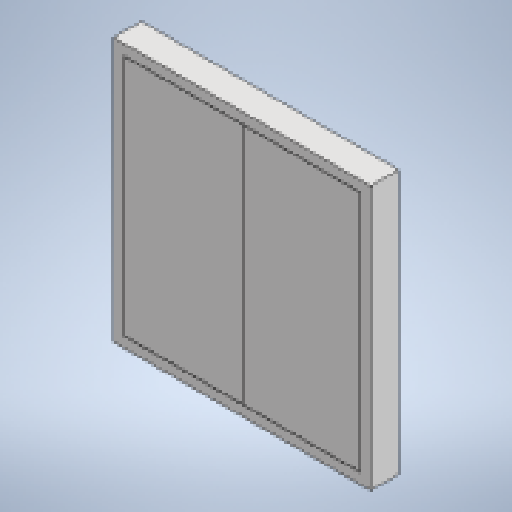
# Autodesk Inventor part: BSH 0 foudation
Saved by Autodesk Inventor 2025 (Build 290162010, 162A)
## iProperties
Created: 2024-08-27
Part Number: BSH 0 foudation
Material: Generic
Document SubType Name: Modeling
Designer: DELL
Density: 1 g/cm^3
Appearance: Default
Author: DELL
Autodesk Inventor part; units mm, degrees
ref_plane "YZ Plane" through (0, 0, 0) normal (1, 0, 0) x (0, 1, 0)
ref_plane "XZ Plane" through (0, 0, 0) normal (0, 1, 0) x (-1, 0, 0)
ref_plane "XY Plane" through (0, 0, 0) normal (0, 0, 1) x (1, 0, 0)
sketch "Sketch1" plane through (0, 0, 0) normal (0, 1, 0) x (-1, 0, 0)
  line L0 (15.7014, 4425) -> (-15.7014, 4425)
  line L1 (4425, 4550) -> (-4425, 4550)
  line L2 (-4425, 4550) -> (-4425, -4550)
  line L3 (-4425, -4550) -> (4425, -4550)
  line L4 (4425, -4550) -> (4425, 4550)
  line L5 (4425, 4550) -> (-4425, -4550) construction
  line L6 (-4425, 4550) -> (4425, -4550) construction
  line L7 (-4825, 4950) -> (4825, 4950)
  line L8 (4825, 4950) -> (4825, -4950)
  line L9 (4825, -4950) -> (-4825, -4950)
  line L10 (-4825, -4950) -> (-4825, 4950)
  point P0 (0, 0)
  point P1 (0, 0)
  dimension "d0" = 8850
  dimension "d1" = 9100
  dimension "d3" = 400
  constraints: 22 end point, 4 parallel, 2 horizontal, 2 midpoint, 2 perpendicular, 1 coincident, 3 other
  measures "d0" distance of L3.end L2.end
  measures "d1" distance of L2.end L1.end
  measures "d3" distance between parallel lines of L1 L7
extrude "Extrusion1" add sketch "Sketch1" along normal blind 650 and the other way blind 400
sketch "Sketch4" plane through (0, -400, 0) normal (0, -1, 0) x (1, 0, 0)
  line L0 (-4825, -4950) -> (4825, -4950) projected
  line L1 (4825, -4950) -> (4825, 4950) projected
  line L2 (4825, 4950) -> (-4825, 4950) projected
  line L3 (-4825, 4950) -> (-4825, -4950) projected
  line L4 (-4425, -4550) -> (-4425, 4550) projected
  line L5 (-4425, 4550) -> (4425, 4550) projected
  line L6 (4425, 4550) -> (4425, -4550) projected
  line L7 (4425, -4550) -> (-4425, -4550) projected
  point P0 (0, 0)
extrude "Extrusion3" add sketch "Sketch4" along normal blind 10 contours L4 L5 L6 L7
sketch "Sketch5" plane through (0, 0, 0) normal (0, 1, 0) x (-1, 0, 0)
  line L0 (-4825, -4950) -> (4825, -4950) projected
  line L1 (4825, -4950) -> (4825, 4950) projected
  line L2 (4825, 4950) -> (-4825, 4950) projected
  line L3 (-4825, 4950) -> (-4825, -4950) projected
  line L4 (4425, 4550) -> (4425, -4550) projected
  line L5 (4425, -4550) -> (-4425, -4550) projected
  line L6 (-4425, -4550) -> (-4425, 4550) projected
  line L7 (-4425, 4550) -> (4425, 4550) projected
  line L8 (5, 4550) -> (5, -4550)
  point P0 (0, 0)
  dimension "d21" = 4420
  constraints: 2 end point, 2 point on line, 1 perpendicular
  measures "d21" distance between parallel lines of L4 L8
extrude "Extrusion4" add sketch "Sketch5" against normal up to surface (400 mm away) contours L4 L5 L8 L7
sketch "Sketch6" plane through (0, 650, 0) normal (0, 1, 0) x (1, 0, 0)
  line L0 (4825, 4950) -> (-4825, 4950) projected
  line L1 (-4825, 4950) -> (-4825, -4950) projected
  line L2 (-4825, -4950) -> (4825, -4950) projected
  line L3 (4825, -4950) -> (4825, 4950) projected
  line L4 (-4425, -4550) -> (-4425, 4550) projected
  line L5 (-4425, 4550) -> (4425, 4550) projected
  line L6 (4425, 4550) -> (4425, -4550) projected
  line L7 (4425, -4550) -> (-4425, -4550) projected
  line L8 (1295, -4950) -> (1295, -4550)
  line L9 (2395, -4950) -> (2395, -4550)
  line L10 (-5, -4550) -> (-5, 4550) projected
  point P0 (0, 0)
  dimension "d24" = 1100
  dimension "d25" = 1300
  constraints: 4 end point, 4 point on line, 2 perpendicular
  measures "d24" distance between parallel lines of L9 L8
  measures "d25" distance between parallel lines of L8 L10
extrude "Extrusion5" cut sketch "Sketch6" against normal blind 10 contours L2 L8 L7 L9
sketch "Sketch7" plane through (1295, 650, 4950) normal (1, 0, 0) x (0, 0, -1)
  line L0 (0, -1050) -> (0, 0) projected
  line L1 (9900, 0) -> (0, 0) projected
  line L2 (9900, -1050) -> (9900, 0) projected
  line L3 (0, -1050) -> (9900, -1050) projected
  line L4 (9500, -1050) -> (400, -1050) projected
  line L5 (9500, -650) -> (9500, -1050) projected
  line L6 (400, -650) -> (9500, -650) projected
  line L7 (400, -1050) -> (400, -650) projected
  line L8 (400, 0) -> (400, -650) projected
  line L9 (400, 0) -> (1200, -150)
  line L10 (1200, -150) -> (1200, -650)
  line L11 (1200, -150) -> (2700, -150)
  line L12 (2700, -150) -> (2700, -650)
  point P0 (4950, -650)
  point P1 (400, -1050)
  dimension "d42" = 10.62
  dimension "d43" = 1500
  dimension "d48" = 800
  dimension "d55" = 900
  constraints: 8 end point, 2 point on line, 1 horizontal, 1 perpendicular, 1 vertical
  measures "d42" angle of L1 L9
  measures "d43" distance of L9.end L11.end
  measures "d48" distance between parallel lines of L10 L8
  measures "d55" distance between parallel lines of L3 L11
extrude "Extrusion6" [suppressed]
sketch "Sketch8" plane through (0, 0, 0) normal (0, 1, 0) x (1, 0, 0)
  circle A0 centre (-2375, -3700) radius 25
  circle A1 centre (-2055, -3700) radius 25
  line L0 (-4425, -4550) -> (-4425, 4550) projected
  line L1 (1295, -4550) -> (-4425, -4550) projected
  point P0 (0, 0)
  dimension "d32" = 50
  dimension "d33" = 2050
  dimension "d34" = 850
  dimension "d35" = 2370
  constraints: 2 centre point, 1 equal radius, 1 horizontal alignment
  measures "d32" diameter of A0
  measures "d33" distance from line of A0.centre L0
  measures "d34" distance from line of L1 A0.centre
  measures "d35" distance from line of A1.centre L0
extrude "Extrusion7" cut sketch "Sketch8" against normal blind 10
sketch "Sketch12" plane through (1295, 0, 2250) normal (0, 0, -1) x (-1, 0, 0)
  line L0 (0, 500) -> (-1100, 500) projected
  line L1 (3645, 0) -> (3695, 0) projected
  line L2 (3325, 0) -> (3375, 0) projected
  line L3 (1300, 0) -> (5720, 0) projected
  line L4 (5720, 0) -> (1300, 0) projected
  line L5 (1300, 0) -> (5720, 0) projected
  line L6 (2850, 0) -> (2850, 200)
  line L7 (2850, 200) -> (0, 200)
  line L8 (0, 200) -> (0, 500)
  line L9 (-1100, 500) -> (-1100, 0)
  line L10 (-1100, 0) -> (2850, 0)
  line L11 (0, 500) -> (1350, 200)
  point P0 (1295, 0)
  point P1 (1300, 0)
  dimension "d49" = 200
  dimension "d50" = 12.529
  dimension "d51" = 1350
  dimension "d54" = 1500
  constraints: 12 end point, 3 perpendicular, 1 collinear, 1 point on line, 1 vertical, 2 other
  measures "d49" distance of L6.start L6.end
  measures "d50" angle of L7 L11
  measures "d51" distance from line of L8 L11.end
  measures "d54" distance of L6.end L11.end
extrude "Extrusion10" [suppressed]
body "Solid1"
